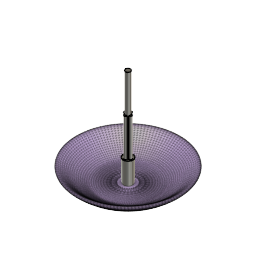
plate (Autodesk Fusion 360 design; units mm, degrees)
Autodesk Fusion 360 part; units mm, degrees
other "Base Mesh Feature1"
sketch "Sketch1" plane through (0, 0, 0) normal (0, 0, 1) x (1, 0, 0)
  circle A0 centre (0, 0) radius 0.6594
  constraint coincident A0.centre origin
extrude "Extrude1" add sketch "Sketch1" along normal blind 15.0114
extrude "Extrude2" cut 1 faces at (0.1099, 0.1903, 0) along direction (0, 0, 1) blind 1.778
sketch "Sketch2" plane through (0, 0, 15.0114) normal (0, 0, 1) x (-1, 0, 0)
  circle A0 centre (0, 0) radius 0.6594
  circle A1 centre (0, 0) radius 0.3417
  constraint coincident A0.centre A1.centre
extrude "Extrude3" cut sketch "Sketch2" against normal blind 5.0038
extrude "Extrude4" cut 1 faces at (0.551, 0.0328, 10.0076) along direction (0, 0, -1) blind 5.0038
sketch "Sketch3" plane through (0, 0, 5.0038) normal (0, 0, 1) x (-1, 0, 0)
  circle A0 centre (0, 0) radius 0.3417
  circle A1 centre (0, 0) radius 0.6594
  circle A2 centre (0.3417, 0.0005) radius 0.1909
  circle A3 centre (-0.3417, -0.0014) radius 0.1956
  circle A4 centre (-0.0012, 0.3417) radius 0.186
  circle A5 centre (-0.0012, -0.3417) radius 0.1876
  constraint coincident A0 A2.centre
  constraint coincident A0 A3.centre
  constraint coincident A0 A4.centre
  constraint coincident A0 A5.centre
extrude "Extrude5" add sketch "Sketch3" along normal blind 5.0038 contours A0 A2 | A0 A4 | A0 A5 | A0 A3 picked at (0.4016, 0.0342) picked at (-0.0388, 0.3986) picked at (-0.0392, -0.399) picked at (-0.4011, -0.0418)
sketch "Sketch5" plane through (0, 0, 0) normal (0, 0, 1) x (1, 0, 0)
  circle A0 centre (3.8, -0.0073) radius 0.381
  dimension "d14" = 0.762
  measures "d14" diameter of A0
